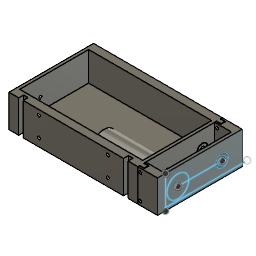
Untitled (Autodesk Fusion 360 design; units mm, degrees)
Autodesk Fusion 360 part; units mm, degrees
note: some values were not read from the file. Chosen so that the rebuilt part matches the saved one: which bodies a step acts on. Set by a fixed rule: which sketch regions a step uses.
sketch "Sketch1" plane through (0, 0, 0) normal (0, 1, 0) x (1, 0, 0)
  line L0 (62.5, 35) -> (-62.5, 35)
  line L1 (-62.5, 35) -> (-62.5, -35)
  line L2 (-62.5, -35) -> (62.5, -35)
  line L3 (62.5, -35) -> (62.5, 35)
  line L4 (62.5, 35) -> (-62.5, -35) construction
  line L5 (-62.5, 35) -> (62.5, -35) construction
  line L6 (-62.5, -35) -> (-10.5, -35)
  line L7 (-10.5, -35) -> (-10.5, -10)
  line L8 (-10.5, -10) -> (-62.5, -10)
  line L9 (-62.5, -10) -> (-62.5, -35)
  line L10 (62.5, -35) -> (10.5, -35)
  line L11 (10.5, -35) -> (10.5, -10)
  line L12 (10.5, -10) -> (62.5, -10)
  line L13 (62.5, -10) -> (62.5, -35)
  line L14 (-65.5, -38) -> (65.5, -38)
  line L15 (65.5, -38) -> (65.5, 43)
  line L16 (-65.5, 43) -> (-65.5, -38)
  line L17 (65.5, 43) -> (-65.5, 43)
  dimension "d1" = 125
  dimension "d2" = 70
  dimension "d3" = 52
  dimension "d4" = 25
  dimension "d5" = 52
  dimension "d6" = 25
  constraint horizontal L0
  constraint perpendicular L0 L1
  constraint parallel L0 L2
  constraint parallel L1 L3
  constraint coincident L4 origin
  constraint coincident L5 origin
  constraint horizontal L6
  constraint vertical L7
  constraint horizontal L8
  constraint vertical L9
  constraint horizontal L10
  constraint vertical L11
  constraint horizontal L12
  constraint vertical L13
  constraint perpendicular L15 L17
  measures "d1" distance of L1.end L2.end
  measures "d2" distance of L0.end L1.end
  measures "d3" distance of L1.end L6.end
  measures "d4" distance of L1.end L8.end
  measures "d5" distance of L2.end L10.end
  measures "d6" distance of L2.end L12.end
extrude "Extrude1" add sketch "Sketch1" along normal blind 25 contours L2 L3 L10 L11 L12 L13 | L1 L2 L6 L7 L8 L9 makes body 1 at (-27.8333, 8.3333, 10) makes body 2 at (45.1667, 0, 26.6667)
sketch "Sketch2" plane through (62.5, 0, 0) normal (1, 0, 0) x (0, 0, -1)
  circle A0 centre (-22.5, 12.5) radius 12.5
  circle A1 centre (-22.5, 12.5) radius 3.5
  circle A2 centre (-22.5, 12.5) radius 3.65
  circle A3 centre (-22.5, 12.5) radius 2
  circle A4 centre (-14, 12.5) radius 1.5
  circle A5 centre (-31, 12.5) radius 1.5
  line L0 (-35, 25) -> (-10, 25)
  line L1 (-10, 25) -> (-10, 0)
  line L2 (-10, 0) -> (-35, 0)
  line L3 (-35, 0) -> (-35, 25)
  dimension "d45" = 7
  dimension "d46" = 7.3
  dimension "d47" = 4
  dimension "d49" = 3
  constraint concentric A0 A1
  constraint concentric A1 A2
  constraint concentric A0 A3
  constraint horizontal L0
  constraint vertical L1
  constraint horizontal L2
  constraint vertical L3
  measures "d45" diameter of A1
  measures "d46" diameter of A2
  measures "d47" diameter of A3
  measures "d49" diameter of A4
extrude "Extrude2" cut sketch "Sketch2" against normal blind 140 contours A0 L1 L2 | A0 L0 L1 | A0 L0 L3 | A0 L2 L3 bodies 1 2
extrude "Extrude3" add sketch "Sketch1" along normal blind 30 separate body makes body 3
extrude "Extrude4" add sketch "Sketch2" along normal blind 2.5 contours A1 bodies 2
extrude "Extrude5" add sketch "Sketch2" along normal blind 12 contours A3 bodies 2
extrude "Extrude6" add sketch "Sketch2" along normal blind -125 and the other way blind 137 contours A3 bodies 1
extrude "Extrude7" add sketch "Sketch2" along normal blind -125 and the other way blind 127.5 contours A1 bodies 1
extrude "Extrude8" cut sketch "Sketch2" along normal blind -128 and the other way blind -3 contours A1 | A2 | A3 bodies 3
extrude "Extrude9" add sketch "Sketch1" against normal blind 3 bodies 3
extrude "Extrude10" add sketch "Sketch1" along normal blind -3 and the other way blind -0.5 contours L0 L1 L2 L3 L7 L8 L11 L12 | L2 L3 L10 L11 L12 L13 | L1 L2 L6 L7 L8 L9 bodies 3
extrude "Extrude11" cut sketch "Sketch2" along normal mid plane 410 contours A4 | A5 bodies 3
sketch "Sketch4" plane through (0, 30, 0) normal (0, 1, 0) x (-1, 0, 0)
  line L0 (62.5, -35) -> (-62.5, -35)
  line L1 (-62.5, -35) -> (-62.5, 35)
  line L2 (-62.5, 35) -> (62.5, 35)
  line L3 (62.5, 35) -> (62.5, -35)
  line L4 (65.5, -43) -> (65.5, 38)
  line L5 (65.5, 38) -> (-65.5, 38)
  line L6 (-65.5, 38) -> (-65.5, -43)
  line L7 (65.5, 38) -> (65.5, 43)
  line L8 (-65.5, 38) -> (-65.5, 43)
  line L9 (55.5, 38) -> (55.5, 43)
  line L10 (55.5, 38) -> (51, 38)
  line L11 (51, 38) -> (51, 43)
  line L12 (0, 38) -> (0, 43)
  line L13 (-51, 38) -> (-51, 43)
  line L14 (-55.5, 38) -> (-55.5, 43)
  line L15 (-55.5, 38) -> (-51, 38)
  line L16 (65.5, 43) -> (55.5, 43)
  line L17 (51, 43) -> (-51, 43)
  line L18 (-55.5, 43) -> (-65.5, 43)
  line L19 (51.4, 38.4) -> (51.4, 43.4)
  line L20 (55.1, 38.4) -> (51.4, 38.4)
  line L21 (55.1, 38.4) -> (55.1, 43.4)
  line L22 (55.1, 43.4) -> (65.5, 43.4)
  line L23 (65.5, 43.4) -> (65.5, 46.4)
  line L24 (-65.5, 46.4) -> (-65.5, 43.4)
  line L25 (51.4, 43.4) -> (-51.4, 43.4)
  line L26 (-55.1, 38.4) -> (-55.1, 43.4)
  line L27 (-55.1, 38.4) -> (-51.4, 38.4)
  line L28 (-51.4, 38.4) -> (-51.4, 43.4)
  line L29 (-55.1, 43.4) -> (-55.2725, 43.4)
  line L30 (-55.2725, 43.4) -> (-65.5, 43.4)
  line L31 (65.5, 46.4) -> (65.5, 66)
  line L32 (62.5, 46.4) -> (62.5, 66)
  line L33 (65.5, 66) -> (62.5, 66)
  line L34 (50.8636, 46.4) -> (50.8636, 66)
  line L35 (53.8636, 46.4) -> (53.8636, 66)
  line L36 (53.8636, 66) -> (50.8636, 66)
  line L37 (39.2273, 46.4) -> (39.2273, 66)
  line L38 (42.2273, 46.4) -> (42.2273, 66)
  line L39 (42.2273, 66) -> (39.2273, 66)
  line L40 (27.5909, 46.4) -> (27.5909, 66)
  line L41 (30.5909, 46.4) -> (30.5909, 66)
  line L42 (30.5909, 66) -> (27.5909, 66)
  line L43 (15.9545, 46.4) -> (15.9545, 66)
  line L44 (18.9545, 46.4) -> (18.9545, 66)
  line L45 (18.9545, 66) -> (15.9545, 66)
  line L46 (4.3182, 46.4) -> (4.3182, 66)
  line L47 (7.3182, 46.4) -> (7.3182, 66)
  line L48 (7.3182, 66) -> (4.3182, 66)
  line L49 (-7.3182, 46.4) -> (-7.3182, 66)
  line L50 (-4.3182, 46.4) -> (-4.3182, 66)
  line L51 (-4.3182, 66) -> (-7.3182, 66)
  line L52 (-18.9545, 46.4) -> (-18.9545, 66)
  line L53 (-15.9545, 46.4) -> (-15.9545, 66)
  line L54 (-15.9545, 66) -> (-18.9545, 66)
  line L55 (-30.5909, 46.4) -> (-30.5909, 66)
  line L56 (-27.5909, 46.4) -> (-27.5909, 66)
  line L57 (-27.5909, 66) -> (-30.5909, 66)
  line L58 (-42.2273, 46.4) -> (-42.2273, 66)
  line L59 (-39.2273, 46.4) -> (-39.2273, 66)
  line L60 (-39.2273, 66) -> (-42.2273, 66)
  line L61 (-53.8636, 46.4) -> (-53.8636, 66)
  line L62 (-50.8636, 46.4) -> (-50.8636, 66)
  line L63 (-50.8636, 66) -> (-53.8636, 66)
  line L64 (-65.5, 46.4) -> (-65.5, 66)
  line L65 (-62.5, 46.4) -> (-62.5, 66)
  line L66 (-62.5, 66) -> (-65.5, 66)
  line L67 (62.5, 46.4) -> (53.8636, 46.4)
  line L68 (50.8636, 46.4) -> (42.2273, 46.4)
  line L69 (39.2273, 46.4) -> (30.5909, 46.4)
  line L70 (27.5909, 46.4) -> (18.9545, 46.4)
  line L71 (15.9545, 46.4) -> (7.3182, 46.4)
  line L72 (4.3182, 46.4) -> (-4.3182, 46.4)
  line L73 (-7.3182, 46.4) -> (-15.9545, 46.4)
  line L74 (-18.9545, 46.4) -> (-27.5909, 46.4)
  line L75 (-30.5909, 46.4) -> (-39.2273, 46.4)
  line L76 (-42.2273, 46.4) -> (-50.8636, 46.4)
  line L77 (-53.8636, 46.4) -> (-62.5, 46.4)
  line L78 (-65.5, -43) -> (65.5, -43)
  dimension "d52" = 5
  dimension "d53" = 5
  dimension "d54" = 10
  dimension "d57" = 3
  dimension "d58" = -3
  dimension "d61" = -128
  dimension "d62" = 0
  constraint coincident L4.end L5.start
  constraint perpendicular L5 L7
  constraint coincident L5.end L6.start
  constraint perpendicular L5 L8
  constraint coincident L5 L10.end
  constraint midpoint L5 L12.start
  constraint symmetric L9.start L12 L14.start
  constraint symmetric L9.end L12 L14.end
  constraint symmetric L10.end L12 L13.start
  constraint symmetric L11.end L12 L13.end
  constraint perpendicular L9 L16
  constraint perpendicular L13 L17
  constraint perpendicular L8 L18
  constraint perpendicular L22 L23
  constraint perpendicular L8 L77
  constraint perpendicular L18 L24
  constraint perpendicular L19 L25
  constraint symmetric L12 L19.start L27.end
  constraint symmetric L12 L20.start L26.start
  constraint symmetric L12 L21.end L26.end
  constraint symmetric L12 L19.end L25.end
  constraint perpendicular L26 L29
  constraint perpendicular L24 L30
  constraint perpendicular L31 L67
  constraint perpendicular L32 L33
  constraint collinear L67 L68
  constraint collinear L68 L69
  constraint collinear L69 L70
  constraint collinear L70 L71
  constraint collinear L71 L72
  constraint collinear L72 L73
  constraint collinear L73 L74
  constraint collinear L74 L75
  constraint collinear L75 L76
  constraint collinear L76 L77
  measures "d52" distance of L4.end L7.end
  measures "d53" distance of L5.end L8.end
  measures "d54" distance of L4.end L9.start
  measures "d57" distance of L22.end L23.end
extrude "Extrude12" add sketch "Sketch4" against normal blind 33 contours L5 L7 L9 L16 | L5 L8 L14 L18 | L5 L11 L12 L17 | L5 L12 L13 L17 bodies 3
extrude "Extrude13" add sketch "Sketch4" against normal blind 33 separate body contours L19 L20 L21 L22 L23 L24 L25 L26 L27 L28 L29 L30 L31 L32 L33 L34 L35 L36 L37 L38 L39 L40 L41 L42 L43 L44 L45 L46 L47 L48 L49 L50 L51 L52 L53 L54 L55 L56 L57 L58 L59 L60 L61 L62 L63 L64 L65 L66 L67 L68 L69 L70 L71 L72 L73 L74 L75 L76 L77 makes body 4
sketch "Sketch5" plane through (0, 0, 35) normal (0, 0, -1) x (-1, 0, 0)
  line L0 (-62.5, 0.5) -> (62.5, 0.5)
  line L1 (62.5, 0.5) -> (62.5, 30)
  line L2 (62.5, 30) -> (-62.5, 30)
  line L3 (-62.5, 30) -> (-62.5, 0.5)
  circle A0 centre (-35, 25) radius 2.5
  circle A1 centre (-35, 25) radius 1.5
  circle A2 centre (-35, 5) radius 1.5
  circle A3 centre (-35, 5) radius 2.5
  circle A4 centre (35, 25) radius 1.5
  circle A5 centre (35, 25) radius 2.5
  circle A6 centre (35, 5) radius 1.5
  circle A7 centre (35, 5) radius 2.5
  dimension "d67" = 5
  dimension "d68" = 3
  dimension "d73" = 5
  dimension "d74" = 5
  dimension "d75" = 5
  constraint concentric A0 A1
  measures "d67" diameter of A0
  measures "d68" diameter of A1
  measures "d73" diameter of A3
  measures "d74" diameter of A7
  measures "d75" diameter of A5
extrude "Extrude14" cut sketch "Sketch5" against normal blind 23 contours A1 | A2 | A4 | A6 bodies 3 4
extrude "Extrude15" cut sketch "Sketch5" against normal blind 3 contours A0 | A3 | A5 | A7 bodies 3
sketch "Sketch6" plane through (65.5, 0, 0) normal (1, 0, 0) x (0, 0, -1)
  line L0 (-46.4, 30) -> (-66, 30)
  line L1 (-66, 30) -> (-66, -3)
  line L2 (-66, -3) -> (-46.4, -3)
  line L3 (-46.4, -3) -> (-46.4, 30)
  line L4 (-46.4, 30) -> (-66, -3)
  constraint coincident L0.start L3.end
  constraint coincident L1.end L2.start
extrude "Extrude16" cut sketch "Sketch6" against normal blind 131 contours L0 L1 L4 bodies 4
sketch "Sketch8" plane through (0, 30, 0) normal (0, 1, 0) x (-1, 0, 0)
  line L0 (62.5, -35) -> (-62.5, -35)
  line L1 (-62.5, -35) -> (-62.5, 35)
  line L2 (-62.5, 35) -> (62.5, 35)
  line L3 (62.5, 35) -> (62.5, -35)
  line L4 (65.5, -43) -> (65.5, 43)
  line L5 (65.5, 43) -> (55.5, 43)
  line L6 (55.5, 43) -> (55.5, 38)
  line L7 (55.5, 38) -> (51, 38)
  line L8 (51, 38) -> (51, 43)
  line L9 (51, 43) -> (-51, 43)
  line L10 (-51, 43) -> (-51, 38)
  line L11 (-51, 38) -> (-55.5, 38)
  line L12 (-55.5, 38) -> (-55.5, 43)
  line L13 (-55.5, 43) -> (-65.5, 43)
  line L14 (-65.5, 43) -> (-65.5, -43)
  line L15 (-85.5, 43) -> (-65.5, 43)
  line L16 (-85.5, -43) -> (-65.5, -43)
  line L17 (-82.5, -35) -> (-65.5, -35)
  line L18 (-82.5, 35) -> (-82.5, -35)
  line L19 (-65.5, 35) -> (-82.5, 35)
  line L20 (-65.5, 43) -> (-65.5, 41.4)
  line L21 (-65.5, 41) -> (-70, 41)
  line L22 (-70, 41) -> (-70, 37)
  line L23 (-70, 37) -> (-65.5, 37)
  line L24 (-65.5, 35) -> (-65.5, 36.6)
  line L25 (-65.5, 41.4) -> (-70.4, 41.4)
  line L26 (-70.4, 41.4) -> (-70.4, 36.6)
  line L27 (-70.4, 36.6) -> (-65.5, 36.6)
  line L28 (-65.5, 37) -> (-65, 37)
  line L29 (-65, 37) -> (-65, 41)
  line L30 (-65, 41) -> (-65.5, 41)
  line L31 (-65.5, -43) -> (65.5, -43)
  line L32 (-85.5, 43) -> (-85.5, -43)
  line L33 (-75.5, 0) -> (-52.9266, 0)
  line L34 (-65.5, -41) -> (-70, -41)
  line L35 (-65, -41) -> (-65.5, -41)
  line L36 (-65, -37) -> (-65, -41)
  line L37 (-65.5, -37) -> (-65, -37)
  line L38 (-70, -37) -> (-65.5, -37)
  line L39 (-70, -41) -> (-70, -37)
  line L40 (-70.4, -41.4) -> (-70.4, -36.6)
  line L41 (-70.4, -36.6) -> (-65.5, -36.6)
  line L42 (-65.5, -35) -> (-65.5, -36.6)
  line L43 (-65.5, -41.4) -> (-70.4, -41.4)
  line L44 (-65.5, -43) -> (-65.5, -41.4)
  dimension "d83" = 0.4
  constraint coincident L13.end L14.start
  constraint perpendicular L14 L15
  constraint coincident L14.end L16.end
  constraint perpendicular L14 L16
  constraint perpendicular L18 L19
  constraint coincident L14 L19.start
  constraint coincident L14 L21.start
  constraint perpendicular L20 L21
  constraint perpendicular L21 L22
  constraint coincident L14 L23.end
  constraint perpendicular L14 L23
  constraint perpendicular L24 L28
  constraint perpendicular L28 L29
  constraint perpendicular L20 L30
  constraint perpendicular L14 L33
  constraint symmetric L13.end L33 L14.end
  constraint symmetric L19.start L33 L17.end
  constraint symmetric L21.start L33 L34.start
  constraint symmetric L21.end L33 L34.end
  constraint symmetric L22.end L33 L38.start
  constraint symmetric L23.end L33 L37.start
  constraint symmetric L20.end L33 L43.start
  constraint symmetric L25.end L33 L40.start
  constraint symmetric L26.end L33 L40.end
  constraint symmetric L24.end L33 L41.end
  constraint symmetric L28.end L33 L36.start
  constraint symmetric L29.end L33 L35.start
extrude "Extrude17" add sketch "Sketch8" against normal blind 33 contours L14 L34 L38 L39 | L14 L21 L22 L23 bodies 3
extrude "Extrude18" add sketch "Sketch8" against normal blind 33 separate body contours L14 L15 L16 L17 L18 L19 L20 L24 L25 L26 L27 L32 L40 L41 L42 L43 L44 makes body 5
sketch "Sketch9" plane through (85.5, 0, 0) normal (1, 0, 0) x (0, 0, -1)
  line L0 (43, 30) -> (-43, 30)
  line L1 (-43, 30) -> (-43, -3)
  line L2 (-43, -3) -> (43, -3)
  line L3 (43, -3) -> (43, 30)
  line L4 (-35, 30) -> (-35, -3)
  line L5 (-35, 0) -> (48, 0)
  line L6 (-35, 0) -> (-10, 0)
  circle A0 centre (-22.5, 12.5) radius 2
  circle A1 centre (22.5, 12.5) radius 2.5
  circle A2 centre (-22.5, 12.5) radius 11
  line L7 (-22.5, 12.5) -> (22.5, 12.5)
  circle A3 centre (22.5, 12.5) radius 5
  circle A4 centre (22.5, 12.5) radius 5.5
  dimension "d88" = 4
  dimension "d89" = 22
  dimension "d92" = 5
  dimension "d93" = 10
  dimension "d94" = 0.5
  constraint coincident L0 L4.start
  constraint coincident L2 L4.end
  constraint perpendicular L2 L4
  constraint coincident L4 L5.start
  constraint perpendicular L4 L5
  constraint coincident L5 L6.end
  constraint concentric A0 A2
  constraint coincident A0.centre A2.centre
  constraint coincident A1.centre L7.end
  constraint horizontal L7
  constraint concentric A1 A3
  measures "d88" diameter of A0
  measures "d89" diameter of A2
  measures "d92" diameter of A1
  measures "d93" diameter of A3
extrude "Extrude19" cut sketch "Sketch9" against normal blind 46 contours A1 | A4 bodies 3 5 makes body 7 at (85.5, 13.1667, 23) makes body 6 at (-17, -3, -14)
sketch "Sketch10" plane through (0, 0, 43) normal (0, 0, 1) x (1, 0, 0)
  line L0 (85.5, 30) -> (65.5, 30)
  line L1 (65.5, 30) -> (65.5, -3)
  line L2 (65.5, -3) -> (85.5, -3)
  line L3 (85.5, -3) -> (85.5, 30)
  circle A0 centre (68, 26) radius 1.5
  line L4 (65.5, 30) -> (65.5, -3)
  line L5 (65.5, 13.5) -> (69, 13.5)
  circle A1 centre (68, 1) radius 1.5
  dimension "d95" = 3
  constraint coincident L0.end L1.start
  constraint coincident L1.end L2.start
  constraint midpoint L4 L5.start
  constraint perpendicular L4 L5
  constraint symmetric A0 L5 A1
  measures "d95" diameter of A0
extrude "Extrude20" cut sketch "Sketch10" against normal blind 109 contours A0 | A1 bodies 6 7
hidden bodies 1 4
